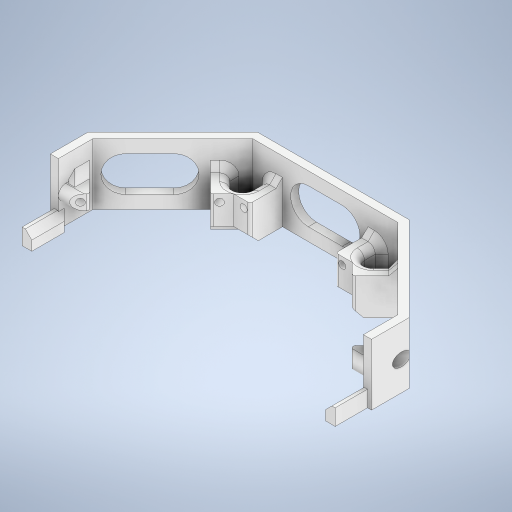
# Autodesk Inventor part: Držák TF-Luna
Saved by Autodesk Inventor 2024 (Build 280153000, 153)
## iProperties
Created: 2023-11-02
Part Number: Držák TF-Luna
Material: Všeobecné
Document SubType Name: Modeling
Designer: 42060
Density: 1 g/cm^3
Appearance: Výchozí
Author: 42060
Autodesk Inventor part; units mm, degrees
ref_plane "YZ Plane" through (0, 0, 0) normal (1, 0, 0) x (0, 1, 0)
ref_plane "XZ Plane" through (0, 0, 0) normal (0, 1, 0) x (-1, 0, 0)
ref_plane "XY Plane" through (0, 0, 0) normal (0, 0, 1) x (1, 0, 0)
sketch "Náčrt1" plane through (0, 0, 0) normal (0, 0, 1) x (1, 0, 0)
  line L0 (0, 0) -> (0, -2.5)
  line L1 (0, -2.5) -> (22.5, -2.5)
  line L2 (22.5, -2.5) -> (47.25, -27.25)
  line L3 (49.75, -26.2145) -> (23.5355, 0)
  line L4 (23.5355, 0) -> (0, 0)
  line L5 (49.75, -26.2145) -> (49.75, -37.923)
  line L6 (49.75, -37.923) -> (47.25, -37.923)
  line L7 (47.25, -37.923) -> (47.25, -27.25)
  dimension "d0" = 2.5
  dimension "d1" = 22.5
  dimension "d2" = 135
  dimension "d50" = 49.75
  dimension "d54" = 2.5
  dimension "d55" = 2.5
  dimension "d80" = 10.673
  constraints: 16 end point, 3 perpendicular, 2 vertical, 1 parallel
  measures "d0" distance of L0.start L0.end
  measures "d1" distance of L0.end L1.end
  measures "d2" angle of L2 L1
  measures "d50" distance between parallel lines of L5 L0
  measures "d54" distance between parallel lines of L2 L3
  measures "d55" distance between parallel lines of L5 L7
  measures "d80" distance from line of L2.end L6
extrude "Vysunutí1" add sketch "Náčrt1" along normal mid plane 19
sketch "Náčrt2" plane through (0, -2.5, 9.5) normal (0, -1, 0) x (1, 0, 0)
  line L0 (22.5, -19) -> (22.5, 0) projected
  line L1 (0, 0) -> (22.5, 0) projected
  line L2 (0, -19) -> (0, 0) projected
  line L3 (22.5, -19) -> (0, -19) projected
  line L4 (13.25, -7.75) -> (15.25, -7.75)
  arc A0 (15.25, -12.25) -> (15.25, -7.75) centre (15.25, -10) ccw
  line L5 (15.25, -12.25) -> (13.25, -12.25)
  line L6 (13.25, -12.25) -> (13.25, -7.75)
  point P0 (0, -9.5)
  dimension "d6" = 2.25
  dimension "d8" = 9
  dimension "d148" = 13.25
  dimension "d149" = 15.25
  constraints: 6 end point, 2 point on circle, 2 tangent, 1 centre point, 1 horizontal, 1 parallel, 1 perpendicular
  measures "d6" radius of A0
  measures "d8" distance from line of L3 A0.centre
  measures "d148" distance between parallel lines of L6 L2
  measures "d149" distance from line of L2 A0.centre
extrude "Vysunutí2" add sketch "Náčrt2" along normal blind 10 contours L4 A0 L5 L6
sketch "Náčrt4" plane through (47.25, -27.25, 9.5) normal (-0.7071068, -0.7071068, 0) x (-0.7071068, 0.7071068, 0)
  line L0 (25.7518, 7.75) -> (27.7518, 7.75)
  arc A0 (27.7518, 7.75) -> (27.7518, 12.25) centre (27.7518, 10) ccw
  line L1 (27.7518, 12.25) -> (25.7518, 12.25)
  line L2 (25.7518, 12.25) -> (25.7518, 7.75)
  line L3 (0, 19) -> (0, 0) projected
  line L4 (35.0018, 0) -> (0, 0) projected
  line L5 (35.0018, 19) -> (35.0018, 0) projected
  line L6 (0, 19) -> (35.0018, 19) projected
  line L7 (41.5425, 12.25) -> (41.5425, 7.75) projected
  line L8 (12.5018, 19) -> (12.5018, 0) construction
  line L9 (-0.7482, 12.25) -> (-0.7482, 7.75)
  line L10 (-0.7482, 7.75) -> (-5.2482, 7.75)
  line L11 (-5.2482, 7.75) -> (-5.2482, 12.25)
  line L12 (-5.2482, 12.25) -> (-0.7482, 12.25)
  point P0 (52.6795, 9.5)
  point P1 (30.0018, 10)
  point P2 (-2.7482, 10)
  dimension "d22" = 15.25
  dimension "d33" = 2.25
  dimension "d39" = 5
  dimension "d150" = 13.25
  constraints: 16 end point, 4 perpendicular, 3 point on circle, 3 symmetric about line, 2 horizontal, 2 point on line, 2 tangent, 1 centre point, 1 horizontal alignment, 1 parallel, 1 vertical
  measures "d22" distance from line of L8 A0.centre
  measures "d33" radius of A0
  measures "d39" distance from line of L5 point (30.002, 10)
  measures "d150" distance between parallel lines of L8 L2
extrude "Vysunutí3" add sketch "Náčrt4" along normal blind 10 contours L2 L1 A0 L0 | L9 L10 L11 L12
sketch "Náčrt8" plane through (49.75, -37.923, 9.5) normal (1, 0, 0) x (0, 0, -1)
  line L0 (7.75, 8.173) -> (12.25, 8.173) projected
  line L1 (7.75, 6.962) -> (7.75, 8.173) projected
  line L2 (12.25, 6.962) -> (7.75, 6.962) projected
  line L3 (12.25, 8.173) -> (12.25, 6.962) projected
  line L4 (12.25, 5.7509) -> (7.75, 5.7509) projected
  line L5 (12.25, 6.962) -> (12.25, 5.7509) projected
  line L6 (12.25, 6.962) -> (7.75, 6.962) projected
  line L7 (7.75, 6.962) -> (7.75, 5.7509) projected
  point P0 (9.5, 37.923)
extrude "Vysunutí7" cut sketch "Náčrt8" along normal through all
sketch "Náčrt10" plane through (13.25, -2.5, 1.75) normal (0, 0, 1) x (1, 0, 0)
  line L0 (2, -10) -> (0, -10) projected
  line L1 (2, -10) -> (4.25, -10) projected
  line L2 (5.7145, -10.6066) -> (7.3055, -12.1976) projected
  line L3 (8.7197, -13.6118) -> (7.3055, -12.1976) projected
  line L4 (4.25, -10) -> (5.1079, -10)
  line L5 (5.1079, -10) -> (5.7145, -10.6066)
  circle A0 centre (7.0345, -5.3488) radius 2.7845
  line L6 (4.25, 0) -> (4.25, -10) projected
  line L7 (12.7855, -3.5355) -> (5.7145, -10.6066) projected
  line L8 (4.25, -5.3488) -> (2, -5.3488)
  line L9 (2, 0) -> (2, -10) projected
  line L10 (9.0034, -7.3177) -> (10.5944, -8.9087)
  line L11 (14.3765, -5.1265) -> (7.3055, -12.1976) projected
  line L12 (5.1079, -10) -> (5.9689, -7.9213) construction
  point P0 (-13.25, 2.5)
  dimension "d70" = 112.5
  constraints: 10 end point, 4 point on line, 3 point on circle, 2 horizontal, 2 tangent, 1 centre point, 1 collinear, 1 equal length, 1 perpendicular
  measures "d70" angle of L4 L12
extrude "Vysunutí9" add sketch "Náčrt10" against normal up to surface (4.5 mm away) contours L9 L8 L6 L1 | L6 A0 L7 L5 L4 | L7 L10 L11 L2
sketch "Náčrt6" plane through (47.25, -27.25, 9.5) normal (-0.7071068, -0.7071068, 0) x (-0.7071068, 0.7071068, 0)
  arc A0 (12.599, 8.2595) -> (12.599, 10.7405) centre (17.7518, 9.5) ccw
  arc A1 (12.4046, 10.7405) -> (12.4046, 8.2595) centre (7.2518, 9.5) ccw
  line L0 (0, 19) -> (0, 0) projected
  line L1 (25.7518, 12.25) -> (25.7518, 7.75) projected
  line L2 (-0.7482, 7.75) -> (-0.7482, 12.25) projected
  line L3 (17.7518, 9.5) -> (25.7518, 9.5) construction
  line L4 (7.2518, 9.5) -> (-0.7482, 9.5) construction
  arc A2 (12.599, 8.2595) -> (12.4046, 8.2595) centre (12.5018, 8.2361) ccw
  arc A3 (12.4046, 10.7405) -> (12.599, 10.7405) centre (12.5018, 10.7639) ccw
  arc A4 (12.5018, 7.8606) -> (12.5018, 11.1394) centre (17.7518, 9.5) ccw
  arc A5 (12.5018, 11.1394) -> (12.5018, 7.8606) centre (7.2518, 9.5) ccw
  line L5 (17.7518, 4) -> (7.2518, 4)
  line L6 (17.7518, 15) -> (7.2518, 15)
  point P0 (52.6795, 9.5)
  point P1 (12.5018, 10.2263)
  point P2 (12.5018, 8.7737)
  point P3 (0, 9.5)
  point P4 (12.599, 10.7405)
  point P5 (12.4046, 8.2595)
  point P6 (12.599, 8.2595)
  dimension "d44" = 10.6
  dimension "d45" = 10.5
  dimension "d48" = 0.2
  dimension "d114" = 0.2
  constraints: 16 point on circle, 8 end point, 7 tangent, 6 centre point, 3 point on line, 2 equal radius, 2 horizontal alignment, 1 collinear, 1 midpoint, 1 parallel, 1 perpendicular, 1 other
  measures "d44" diameter of A1
  measures "d45" distance of L4.start L3.start
  measures "d48" diameter of A2
  measures "d114" radial gap between concentric circles of A0 A4
extrude "Vysunutí5" cut sketch "Náčrt6" against normal blind 11.5 contours A2 A1 A3 A0 | A5 A4 | A4 L5 A5 | A4 A5 L6
sketch "Náčrt7" plane through (0, -2.5, 9.5) normal (0, -1, 0) x (1, 0, 0)
  arc A0 (0.0972, -10.7405) -> (0.0972, -8.2595) centre (5.25, -9.5) ccw
  line L0 (0, -19) -> (0, 0) projected
  arc A1 (0, -8.3361) -> (0.0972, -8.2595) centre (0, -8.2361) ccw
  arc A2 (0.0972, -10.7405) -> (0, -10.6639) centre (0, -10.7639) ccw
  arc A3 (-0.0972, -8.2595) -> (-0.0972, -10.7405) centre (-5.25, -9.5) ccw
  arc A4 (-0.0972, -8.2595) -> (0, -8.3361) centre (0, -8.2361) ccw
  arc A5 (0, -10.6639) -> (-0.0972, -10.7405) centre (0, -10.7639) ccw
  arc A6 (0, -7.8606) -> (0, -11.1394) centre (-5.25, -9.5) ccw
  arc A7 (0, -11.1394) -> (0, -7.8606) centre (5.25, -9.5) ccw
  line L1 (-5.25, -4) -> (5.25, -4)
  line L2 (-5.25, -15) -> (5.25, -15)
  point P0 (0, -9.5)
  point P1 (0, -9.5)
  point P2 (0, -8.7737)
  point P3 (0, -10.2263)
  point P4 (0, -9.5)
  point P5 (0.0972, -8.2595)
  point P6 (0, -8.3361)
  point P7 (0, -10.6639)
  point P8 (0.0972, -10.7405)
  point P9 (0, -8.1361)
  point P10 (0, -10.8639)
  point P11 (0, -11.1394)
  point P12 (0, -15)
  point P13 (0, -4)
  dimension "d40" = 10.6
  dimension "d41" = 5.25
  dimension "d49" = 0.2
  dimension "d115" = 0.2
  constraints: 20 point on circle, 8 centre point, 6 tangent, 4 end point, 3 symmetric about line, 2 midpoint, 2 point on line, 2 vertical alignment, 1 equal radius, 1 horizontal alignment, 4 other
  measures "d40" diameter of A0
  measures "d41" distance from line of A0.centre L0
  measures "d49" diameter of A1
  measures "d115" radial gap between concentric circles of A3 A6
extrude "Vysunutí4" cut sketch "Náčrt7" against normal blind 11.5 contours A2 L0 A1 A0 | A0 A1 L0 A7 A2 | A5 A3 A4 L0 | A7 L2 L0 | L0 L1 A7
sketch "Náčrt11" plane through (0, 0, -9.5) normal (0, 0, -1) x (-1, 0, 0)
  line L0 (-22.5, -2.5) -> (0, -2.5) projected
  line L1 (-47.25, -27.25) -> (-22.5, -2.5) projected
  line L2 (-26.0355, -6.0355) -> (-22.2534, -9.8177) projected
  arc A0 (-22.2534, -9.8177) -> (-17.5, -7.8488) centre (-20.2845, -7.8488) ccw projected
  line L3 (-17.5, -2.5) -> (-17.5, -7.8488) projected
  line L4 (-13.25, -2.5) -> (-13.25, -12.5) projected
  line L5 (-13.25, -12.5) -> (-18.3579, -12.5) projected
  line L6 (-18.3579, -12.5) -> (-21.9697, -16.1118) projected
  line L7 (-29.0407, -9.0407) -> (-21.9697, -16.1118) projected
  circle A1 centre (-20.9693, -6.1955) radius 1.75
  line L8 (-20.2845, -7.8488) -> (-22.5, -2.5) construction
  point P0 (0, 0)
  dimension "d71" = 3.5
  dimension "d72" = 4
  constraints: 2 end point, 1 centre point, 1 point on line
  measures "d71" diameter of A1
  measures "d72" distance of A1.centre L0.start
extrude "Vysunutí10" add sketch "Náčrt11" against normal up to surface (9 mm away) contours L0 L4 L5 L6 L7 L1 L2 A0 L3
sketch "Náčrt3" plane through (0, -12.5, 9.5) normal (0, -1, 0) x (1, 0, 0)
  arc A0 (15.25, -12.25) -> (15.25, -7.75) centre (15.25, -10) ccw projected
  point P0 (0, -9.5)
  constraints: 1 coincident
hole "Díra1" at (15.25, -12.5, -0.5) direction (0, 1, 0) diameter 2.2 end through all
sketch "Náčrt5" plane through (40.1789, -34.3211, 9.5) normal (-0.7071068, -0.7071068, 0) x (0, 0, -1)
  arc A0 (7.75, -27.7518) -> (12.25, -27.7518) centre (10, -27.7518) ccw projected
  line L0 (12.25, 5.2482) -> (7.75, 5.2482) projected
  line L1 (7.75, 5.2482) -> (7.75, 0.7482) projected
  line L2 (7.75, 0.7482) -> (12.25, 0.7482) projected
  line L3 (12.25, 0.7482) -> (12.25, 5.2482) projected
  line L4 (12.25, 0.7482) -> (12.25, 5.2482) projected
  line L5 (12.25, 5.2482) -> (7.75, 5.2482) projected
  line L6 (19, 1.0355) -> (0, 1.0355) projected
  line L7 (0, 9.3147) -> (0, 1.0355) projected
  line L8 (19, 9.3147) -> (0, 9.3147) projected
  line L9 (19, 1.0355) -> (19, 9.3147) projected
  line L10 (19, -12.5018) -> (0, -12.5018) construction
  point P0 (9.5, -52.6795)
  point P1 (10, 2.7482)
  constraints: 1 coincident, 1 symmetric about line
hole "Díra2" at (20.5555, -14.6976, -0.5) at (42.1222, -36.2643, -0.5) direction (0.7071068, 0.7071068, 0) diameter 2.2 end through all
chamfer "Zkosení3" distance 2.5 angle 45 2 edges at (47.25, -31.4901, 1.75) (47.25, -31.4901, -2.75)
sketch "Náčrt9" plane through (47.25, -34.6721, 1.75) normal (0, 0, 1) x (1, 0, 0)
  line L0 (0, -3.2509) -> (0, 7.4221) projected
  line L1 (0, 0) -> (-3.36, -3.36) projected
  line L2 (0, -3.2509) -> (-3.2509, -3.2509)
  line L3 (-3.2509, -3.2509) -> (-3.4691, -3.2509)
  line L4 (-3.36, -3.36) -> (-6.542, -0.178) projected
  line L5 (0, 7.4221) -> (0, -3.2509) projected
  point P0 (-47.25, 34.6721)
  constraints: 4 end point, 2 horizontal, 2 point on line
extrude "Vysunutí8" add sketch "Náčrt9" against normal up to surface (4.5 mm away) contours L2 L1 L0
extrude "Vysunutí17" cut sketch "Náčrt9" against normal through all contours L1 L4 L3
chamfer "Zkosení4" distance 1.5 angle 45 2 edges at (46, -35.9221, 3) (46, -35.9221, -4)
extrude "Vysunutí11" add sketch "Náčrt11" against normal blind 2.5 contours L0 L3 A0 L2 L1
fillet "Zaoblení2" radius 2.25 1 edges at (19.2189, -10.4213, 1.75)
fillet "Zaoblení1" radius 2.25 2 edges at (45.5154, -37.923, 1.75) (45.5154, -37.923, -2.75)
chamfer "Zkosení5" distance 2 angle 45 6 edges at (28.3336, -8.3336, 1.75) (26.5015, -6.5015, 1.091) (26.0355, -6.0355, -3.75) (14.25, -2.5, 1.75) (16.841, -2.5, 1.091) (17.5, -2.5, -3.75)
sketch "Náčrt12" plane through (0, 0, 9.5) normal (0, 1, 0) x (1, 0, 0)
  circle A0 centre (15.25, 10) radius 1.1 projected
  line L0 (15.25, 12.4249) -> (17.35, 11.2124)
  line L1 (17.35, 11.2124) -> (17.35, 8.7876)
  line L2 (17.35, 8.7876) -> (15.25, 7.5751)
  line L3 (15.25, 7.5751) -> (13.15, 8.7876)
  line L4 (13.15, 8.7876) -> (13.15, 11.2124)
  line L5 (13.15, 11.2124) -> (15.25, 12.4249)
  point P0 (0, 9.5)
  dimension "d81" = 4.2
  constraints: 12 end point, 1 coincident, 1 vertical alignment, 13 other
  measures "d81" distance between parallel lines of L4 L1
extrude "Vysunutí12" [suppressed]
sketch "Náčrt13" plane through (23.5355, 0, -9.5) normal (0.7071068, 0.7071068, 0) x (-0.7071068, 0.7071068, 0)
  circle A0 centre (-8.2855, 9) radius 1.1 projected
  line L0 (-8.2855, 6.5751) -> (-10.3855, 7.7876)
  line L1 (-10.3855, 7.7876) -> (-10.3855, 10.2124)
  line L2 (-10.3855, 10.2124) -> (-8.2855, 11.4249)
  line L3 (-8.2855, 11.4249) -> (-6.1855, 10.2124)
  line L4 (-6.1855, 10.2124) -> (-6.1855, 7.7876)
  line L5 (-6.1855, 7.7876) -> (-8.2855, 6.5751)
  line L6 (-38.7855, 6.5751) -> (-40.8855, 7.7876)
  line L7 (-40.8855, 7.7876) -> (-40.8855, 10.2124)
  line L8 (-40.8855, 10.2124) -> (-38.7855, 11.4249)
  line L9 (-38.7855, 11.4249) -> (-36.6855, 10.2124)
  line L10 (-36.6855, 10.2124) -> (-36.6855, 7.7876)
  line L11 (-36.6855, 7.7876) -> (-38.7855, 6.5751)
  circle A1 centre (-38.7855, 9) radius 1.1 projected
  point P0 (16.6421, 9.5)
  point P1 (-8.2855, 9)
  dimension "d84" = 4.2
  dimension "d85" = 4.2
  constraints: 24 end point, 3 coincident, 1 vertical alignment, 26 other
  measures "d84" distance between parallel lines of L4 L1
  measures "d85" distance between parallel lines of L7 L10
extrude "Vysunutí13" [suppressed]
extrude "Vysunutí14" [suppressed]
sketch "Náčrt15" plane through (0, 0, 9.5) normal (0, 1, 0) x (1, 0, 0)
  circle A0 centre (15.25, 10) radius 1.1 projected
  point P0 (0, 9.5)
  constraints: 1 coincident
hole "Díra3" at (15.25, 0, -0.5) direction (0, -1, 0) diameter 4 depth 2
sketch "Náčrt16" plane through (23.5355, 0, -9.5) normal (0.7071068, 0.7071068, 0) x (-0.7071068, 0.7071068, 0)
  circle A0 centre (-8.2855, 9) radius 1.1 projected
  point P0 (16.6421, 9.5)
  constraints: 1 coincident
hole "Díra4" at (29.3943, -5.8588, -0.5) direction (-0.7071068, -0.7071068, 0) diameter 4 depth 2
sketch "Náčrt17" plane through (23.5355, 0, -9.5) normal (0.7071068, 0.7071068, 0) x (-0.7071068, 0.7071068, 0)
  circle A0 centre (-38.7855, 9) radius 1.1 projected
  point P0 (16.6421, 9.5)
  constraints: 2 coincident
hole "Díra5" at (50.961, -27.4255, -0.5) direction (-0.7071068, -0.7071068, 0) diameter 4 depth 6
sketch "Náčrt14" plane through (49.75, -37.923, 9.5) normal (1, 0, 0) x (0, 0, -1)
  line L0 (19, 11.7085) -> (0, 11.7085) projected
  line L1 (19, 11.7085) -> (23, 11.7085)
  line L2 (23, 11.7085) -> (23, 5.7085)
  line L3 (23, 5.7085) -> (21, 5.7085)
  line L4 (21, 5.7085) -> (21, 9.7085)
  line L5 (21, 9.7085) -> (19, 9.7085)
  line L6 (19, 11.7085) -> (19, 0) projected
  point P0 (9.5, 37.923)
  point P1 (11.3812, 11.7085)
  dimension "d105" = 2
  dimension "d106" = 2
  dimension "d107" = 6
  dimension "d108" = 4
  constraints: 10 end point, 3 perpendicular, 1 horizontal, 1 vertical
  measures "d105" distance between parallel lines of L1 L5
  measures "d106" distance between parallel lines of L4 L2
  measures "d107" distance between parallel lines of L1 L3
  measures "d108" distance between parallel lines of L6 L2
extrude "Vysunutí15" [suppressed]
chamfer "Zkosení7" [suppressed]
chamfer "Zkosení1" distance 2.5 angle 45 2 edges at (15.8039, -12.5, -9.5) (20.1638, -14.3059, -9.5)
sketch "Náčrt18" plane through (47.25, -37.923, 9.5) normal (0, -1, 0) x (1, 0, 0)
  line L0 (-23.7145, -19) -> (2.5, -19) projected
  line L1 (1.25, -19) -> (1.25, -14)
  line L2 (1.25, -14) -> (-1.75, -14)
  line L3 (-1.75, -14) -> (-1.75, -19)
  line L4 (2.5, -19) -> (0, -19) projected
  point P0 (-47.25, -9.5)
  dimension "d137" = 3
  dimension "d138" = 5
  constraints: 6 end point, 2 perpendicular, 2 point on line, 1 coincident, 1 midpoint, 1 vertical
  measures "d137" distance of L1.end L2.end
  measures "d138" distance of L2.end L3.end
extrude "Vysunutí16" add sketch "Náčrt18" along normal blind 10
chamfer "Zkosení8" distance 1.75 angle 45 1 edges at (47.25, -37.923, -7)
chamfer "Zkosení9" distance 2 angle 45 1 edges at (45.5, -42.923, -4.5)
fillet "Zaoblení3" radius 0.7 3 edges at (13.25, -12.5, -2.625) (21.9697, -16.1118, -2.625) (40.708, -34.8501, -0.5)
mirror "Zrcadlit1" about plane through (0, 0, 0) normal (1, 0, 0)
